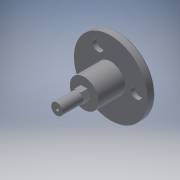
# Autodesk Inventor part: Cutter
Saved by Autodesk Inventor 2019 (Build 230136000, 136)
## iProperties
Created: 2019-03-02
Part Number: Cutter
Material: Generic
Document SubType Name: Modeling
Designer: alarr
Density: 1 g/cm^3
Appearance: Default
Author: alarr
Autodesk Inventor part; units mm, degrees
ref_plane "YZ Plane" through (0, 0, 0) normal (1, 0, 0) x (0, 1, 0)
ref_plane "XZ Plane" through (0, 0, 0) normal (0, 1, 0) x (-1, 0, 0)
ref_plane "XY Plane" through (0, 0, 0) normal (0, 0, 1) x (1, 0, 0)
sketch "Sketch1" plane through (0, 0, 0) normal (0, 0, 1) x (1, 0, 0)
  circle A0 centre (0, 0) radius 45.72
  dimension "d0" = 91.44
  constraints: 1 centre point, 1 coincident
  measures "d0" diameter of A0
extrude "Extrusion1" add sketch "Sketch1" along normal blind 15.24
sketch "Sketch2" plane through (0, 0, 15.24) normal (0, 0, 1) x (1, 0, 0)
  circle A0 centre (0, 0) radius 17.78
  dimension "d3" = 35.56
  constraints: 1 centre point, 1 coincident
  measures "d3" diameter of A0
extrude "Extrusion2" add sketch "Sketch2" along normal blind 33.02
sketch "Sketch3" plane through (0, 0, 48.26) normal (0, 0, 1) x (1, 0, 0)
  line L0 (4.0695, 7.0485) -> (8.1389, 0)
  line L1 (8.1389, 0) -> (4.0695, -7.0485)
  line L2 (4.0695, -7.0485) -> (-4.0695, -7.0485)
  line L3 (-4.0695, -7.0485) -> (-8.1389, 0)
  line L4 (-8.1389, 0) -> (-4.0695, 7.0485)
  line L5 (-4.0695, 7.0485) -> (4.0695, 7.0485)
  point P0 (0, 0)
  point P1 (0, 0)
  dimension "d6" = 14.097
  constraints: 12 end point, 1 coincident, 1 horizontal, 13 other
  measures "d6" distance between parallel lines of L2 L5
extrude "Extrusion3" add sketch "Sketch3" along normal blind 8.382
sketch "Sketch4" plane through (0, 0, 56.642) normal (0, 0, 1) x (1, 0, 0)
  circle A0 centre (0, 0) radius 7.112
  dimension "d9" = 14.224
  constraints: 1 centre point, 1 coincident
  measures "d9" diameter of A0
extrude "Extrusion4" add sketch "Sketch4" along normal blind 25.4
sketch "Sketch5" plane through (0, 0, 82.042) normal (0, 0, 1) x (1, 0, 0)
  circle A0 centre (0, 0) radius 2.413
  dimension "d12" = 4.826
  constraints: 1 centre point, 1 coincident
  measures "d12" diameter of A0
extrude "Extrusion5" cut sketch "Sketch5" against normal up to surface (25.4 mm away)
sketch "Sketch6" plane through (0, 0, 0) normal (0, 0, -1) x (-1, 0, 0)
  circle A0 centre (0, 0) radius 45.72 projected
  circle A1 centre (0, 0) radius 25.4
  dimension "d15" = 50.8
  constraints: 1 centre point, 1 coincident
  measures "d15" diameter of A1
extrude "Extrusion6" cut sketch "Sketch6" against normal blind 5.08
sketch "Sketch7" plane through (0, 0, 0) normal (0, 0, -1) x (-1, 0, 0)
  circle A0 centre (0, 0) radius 17.145
  dimension "d19" = 34.29
  constraints: 1 centre point, 1 coincident
  measures "d19" diameter of A0
extrude "Extrusion7" cut sketch "Sketch7" against normal blind 15.24
fillet "Fillet1" radius 3.175 3 edges at (-45.72, 0, 5.08) (25.4, 0, 5.08) (25.4, 0, 0)
sketch "Sketch8" plane through (0, 0, 15.24) normal (0, 0, -1) x (-1, 0, 0)
  line L0 (8.1389, 0) -> (4.0695, 7.0485) projected
  line L1 (4.0695, -7.0485) -> (8.1389, 0) projected
  line L2 (-4.0695, -7.0485) -> (4.0695, -7.0485) projected
  line L3 (-8.1389, 0) -> (-4.0695, -7.0485) projected
  line L4 (-4.0695, 7.0485) -> (-8.1389, 0) projected
  line L5 (4.0695, 7.0485) -> (-4.0695, 7.0485) projected
  line L6 (4.0695, 7.0485) -> (8.1389, 0)
  line L7 (8.1389, 0) -> (4.0695, -7.0485)
  line L8 (4.0695, -7.0485) -> (-4.0695, -7.0485)
  line L9 (-4.0695, -7.0485) -> (-8.1389, 0)
  line L10 (-8.1389, 0) -> (-4.0695, 7.0485)
  line L11 (-4.0695, 7.0485) -> (4.0695, 7.0485)
  point P0 (0, 0)
  point P1 (0, 0)
  constraints: 12 end point, 1 coincident, 13 other
extrude "Extrusion8" cut sketch "Sketch8" against normal blind 29.845
sketch "Sketch9" plane through (0, 0, 15.24) normal (0, 0, 1) x (1, 0, 0)
  circle A0 centre (31.75, 0) radius 6.985
  circle A1 centre (0, 0) radius 45.72 projected
  line L0 (31.75, 0) -> (45.72, 0) construction
  line L1 (0, 0) -> (31.75, 0) construction
  dimension "d24" = 13.97
  dimension "d25" = 13.97
  constraints: 4 end point, 2 horizontal, 1 centre point, 1 horizontal alignment, 1 other
  measures "d24" diameter of A0
  measures "d25" distance of L0.start L0.end
extrude "Extrusion9" cut sketch "Sketch9" against normal blind 5.08 contours A0
pattern_circular "Circular Pattern1" count 3 over 360 about axis through (0, 0, 15.24) along (0, 0, 1) of "Extrusion9"
body "Solid1"
